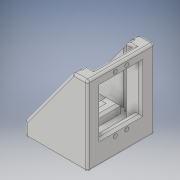
# Autodesk Inventor part: ServoMount2
Saved by Autodesk Inventor 2018 (Build 220112000, 112)
## iProperties
Created: 2018-04-02
Part Number: ServoMount2
Material: Generic
Document SubType Name: Modeling
Designer: anirudh
Density: 1 g/cm^3
Appearance: Default
Author: anirudh
Autodesk Inventor part; units mm, degrees
ref_plane "YZ Plane" through (0, 0, 0) normal (1, 0, 0) x (0, 1, 0)
ref_plane "XZ Plane" through (0, 0, 0) normal (0, 1, 0) x (-1, 0, 0)
ref_plane "XY Plane" through (0, 0, 0) normal (0, 0, 1) x (1, 0, 0)
sketch "Sketch10" plane through (0, 0, 0) normal (0, 1, 0) x (-1, 0, 0)
  line L0 (0, 0) -> (54.4068, 0)
  line L1 (54.4068, 0) -> (54.4068, -58.9534)
  line L2 (54.4068, -58.9534) -> (0, -58.9534)
  line L3 (0, -58.9534) -> (0, 0)
  dimension "d27" = 54.4068
  dimension "d28" = 58.9534
  constraints: 8 end point, 2 parallel, 1 horizontal, 1 perpendicular
  measures "d27" distance of L1.end L2.end
  measures "d28" distance of L0.end L1.end
extrude "Extrusion6" add sketch "Sketch10" along normal blind 76.2
sketch "Sketch12" plane through (0, 0, 0) normal (1, 0, 0) x (0, 0, -1)
  line L0 (58.9534, 0) -> (0, 0) projected
  line L1 (0, 0) -> (58.9534, 0)
  line L2 (58.9534, 0) -> (58.9534, 76.2) projected
  line L3 (0, 0) -> (0, 76.2) projected
  line L4 (29.4767, 20.6375) -> (18.3642, 20.6375)
  line L5 (18.3642, 20.6375) -> (40.5892, 20.6375)
  line L6 (40.5892, 20.6375) -> (40.5892, 60.325)
  line L7 (40.5892, 60.325) -> (18.3642, 60.325)
  line L8 (18.3642, 60.325) -> (18.3642, 20.6375)
  dimension "d39" = 11.1125
  dimension "d40" = 22.225
  constraints: 12 end point, 2 horizontal, 2 parallel, 1 perpendicular
  measures "d39" distance of L4.end L4.start
  measures "d40" distance of L7.end L6.end
extrude "Extrusion7" cut sketch "Sketch12" against normal blind 41.275
sketch "Sketch13" plane through (0, 0, 0) normal (1, 0, 0) x (0, 0, -1)
  line L0 (0, 0) -> (0, 12.7)
  line L1 (0, 12.7) -> (58.9534, 12.7)
  line L2 (0, 68.2752) -> (58.9534, 68.2752)
  line L3 (0, 0) -> (0, 76.2) projected
  line L4 (0, 76.2) -> (58.9534, 76.2)
  line L5 (58.9534, 76.2) -> (58.9534, 68.2752)
  line L6 (58.9534, 68.2752) -> (0, 68.2752)
  line L7 (0, 68.2752) -> (0, 76.2)
  dimension "d43" = 12.7
  constraints: 14 end point, 2 parallel, 2 perpendicular, 1 horizontal
  measures "d43" distance of L0.start L0.end
extrude "Extrusion8" cut sketch "Sketch13" against normal blind 54.4068
sketch "Sketch14" plane through (0, 0, 0) normal (1, 0, 0) x (0, 0, -1)
  line L0 (0, 0) -> (0, 12.7)
  line L1 (0, 0) -> (0, 68.2752) projected
  line L2 (0, 12.7) -> (58.9534, 12.7)
  line L3 (58.9534, 0) -> (58.9534, 68.2752) projected
  line L4 (0, 68.2752) -> (58.9534, 68.2752)
  line L5 (58.9534, 68.2752) -> (58.9534, 12.7)
  line L6 (58.9534, 12.7) -> (0, 12.7)
  line L7 (0, 12.7) -> (0, 68.2752)
  line L8 (18.3642, 60.325) -> (40.5892, 60.325) projected
  line L9 (40.5892, 60.325) -> (40.5892, 20.6375) projected
  line L10 (18.3642, 60.325) -> (40.5892, 60.325)
  line L11 (40.5892, 60.325) -> (40.5892, 20.6375)
  line L12 (40.5892, 20.6375) -> (18.3642, 20.6375)
  line L13 (18.3642, 20.6375) -> (18.3642, 60.325)
  dimension "d47" = 12.7
  constraints: 20 end point, 4 parallel, 3 perpendicular, 2 horizontal, 2 point on line
  measures "d47" distance of L0.start L0.end
extrude "Extrusion9" cut sketch "Sketch14" against normal blind 12.7
sketch "Sketch15" plane through (-54.4068, 0, 0) normal (0, 0, 1) x (1, 0, 0)
  line L0 (41.7068, 12.7) -> (41.7068, 68.2752) projected
  line L1 (0, 0) -> (0, 68.2752) projected
  line L2 (41.7068, 12.7) -> (0, 12.7)
  line L3 (0, 12.7) -> (0, 68.2752)
  line L4 (0, 68.2752) -> (41.7068, 68.2752)
  line L5 (41.7068, 68.2752) -> (41.7068, 12.7)
  point P0 (54.4068, 0)
  constraints: 8 end point, 2 parallel, 1 horizontal, 1 perpendicular
extrude "Extrusion10" cut sketch "Sketch15" against normal blind 12.0142
sketch "Sketch16" plane through (0, 0, -58.9534) normal (0, 0, -1) x (-1, 0, 0)
  line L0 (54.4068, 68.2752) -> (12.7, 68.2752) projected
  line L1 (12.7, 12.7) -> (54.4068, 12.7) projected
  line L2 (12.7, 68.2752) -> (54.4068, 68.2752)
  line L3 (54.4068, 68.2752) -> (54.4068, 12.7)
  line L4 (54.4068, 12.7) -> (12.7, 12.7)
  line L5 (12.7, 12.7) -> (12.7, 68.2752)
  point P0 (0, 0)
  constraints: 8 end point, 2 parallel, 1 horizontal, 1 perpendicular
extrude "Extrusion11" cut sketch "Sketch16" against normal blind 12.0142
sketch "Sketch17" plane through (-54.4068, 0, -58.9534) normal (-1, 0, 0) x (0, 0, 1)
  line L0 (12.0142, 12.7) -> (12.0142, 68.2752) projected
  line L1 (46.9392, 68.2752) -> (46.9392, 12.7) projected
  line L2 (12.0142, 68.2752) -> (46.9392, 68.2752)
  line L3 (46.9392, 68.2752) -> (46.9392, 12.7)
  line L4 (46.9392, 12.7) -> (12.0142, 12.7)
  line L5 (12.0142, 12.7) -> (12.0142, 68.2752)
  point P0 (58.9534, 0)
  constraints: 8 end point, 2 parallel, 1 horizontal, 1 perpendicular
extrude "Extrusion12" cut sketch "Sketch17" against normal blind 6.7818
sketch "Sketch18" plane through (0, 0, 0) normal (0, -1, 0) x (1, 0, 0)
  line L0 (-54.4068, -58.9534) -> (0, -58.9534) projected
  line L1 (0, -58.9534) -> (0, 0) projected
  line L2 (0, 0) -> (-54.4068, 0) projected
  circle A0 centre (-18.034, -52.6034) radius 1.75
  circle A1 centre (-46.7868, -52.6034) radius 1.75
  circle A2 centre (-18.034, -6.35) radius 1.75
  circle A3 centre (-46.7868, -6.35) radius 1.75
  dimension "d61" = 3.5
  dimension "d62" = 3.5
  dimension "d63" = 3.5
  dimension "d64" = 3.5
  constraints: 4 centre point
  measures "d61" diameter of A0
  measures "d62" diameter of A1
  measures "d63" diameter of A2
  measures "d64" diameter of A3
extrude "Extrusion13" cut sketch "Sketch18" against normal blind 12.7
sketch "Sketch21" plane through (-12.7, 0, 0) normal (1, 0, 0) x (0, 0, -1)
  circle A0 centre (24.4348, 64.9986) radius 1.75
  circle A1 centre (34.5186, 64.9986) radius 1.75
  circle A2 centre (24.4348, 15.9639) radius 1.75
  circle A3 centre (34.5186, 15.9639) radius 1.75
  point P0 (0, 0)
  point P1 (18.3642, 20.6375)
  point P2 (18.3642, 60.325)
  dimension "d82" = 3.5
  dimension "d83" = 3.5
  dimension "d84" = 3.5
  dimension "d85" = 3.5
  constraints: 4 centre point
  measures "d82" diameter of A0
  measures "d83" diameter of A1
  measures "d84" diameter of A2
  measures "d85" diameter of A3
extrude "Extrusion15" cut sketch "Sketch21" against normal blind 15.24
sketch "Sketch27" plane through (-12.7, 68.2752, -12.0142) normal (0, 1, 0) x (1, 0, 0)
  line L0 (-28.575, 6.35) -> (-28.575, 28.575) projected
  line L1 (-28.575, 6.35) -> (-5.08, 6.35)
  line L2 (-5.08, 28.575) -> (-28.575, 28.575)
  line L3 (-28.575, 28.575) -> (-28.575, 6.35)
  line L4 (-34.925, 0) -> (-34.925, 34.925) projected
  line L5 (-5.08, 0) -> (-34.925, 0)
  line L6 (-34.925, 0) -> (-34.925, 34.925)
  line L7 (-34.925, 34.925) -> (-5.08, 34.925)
  line L8 (-5.08, 0) -> (-34.925, 0)
  line L9 (-34.925, 0) -> (-34.925, 34.925)
  line L10 (-34.925, 34.925) -> (-5.08, 34.925)
  line L11 (-5.08, 34.925) -> (-5.08, 28.575)
  line L12 (-5.08, 28.575) -> (-28.575, 28.575)
  line L13 (-28.575, 28.575) -> (-28.575, 6.35)
  line L14 (-28.575, 6.35) -> (-5.08, 6.35)
  line L15 (-5.08, 6.35) -> (-5.08, 0)
  point P0 (12.7, -12.0142)
  constraints: 28 end point, 7 equal length, 3 perpendicular, 2 horizontal
extrude "Extrusion18" cut sketch "Sketch27" against normal blind 47.6504
sketch "Sketch28" plane through (-12.7, 68.2752, -12.0142) normal (0, 1, 0) x (1, 0, 0)
  line L0 (-28.575, 28.575) -> (-28.575, 6.35) projected
  line L1 (-5.08, 28.575) -> (-28.575, 28.575) projected
  line L2 (-28.575, 6.35) -> (-5.08, 6.35)
  line L3 (-5.08, 6.35) -> (-5.08, 28.575)
  line L4 (-5.08, 28.575) -> (-28.575, 28.575)
  line L5 (-28.575, 28.575) -> (-28.575, 6.35)
  point P0 (12.7, -12.0142)
  constraints: 8 end point, 2 parallel, 1 horizontal, 1 perpendicular
extrude "Extrusion19" cut sketch "Sketch28" against normal blind 7.9502
sketch "Sketch29" plane through (-12.7, 68.2752, -12.0142) normal (0, 1, 0) x (1, 0, 0)
  line L0 (-5.08, 34.925) -> (-5.08, 28.575) projected
  line L1 (0, 0) -> (-34.925, 0) projected
  line L2 (-5.08, 34.925) -> (0, 34.925)
  line L3 (0, 34.925) -> (0, 0)
  line L4 (0, 0) -> (-5.08, 0)
  line L5 (-5.08, 0) -> (-5.08, 34.925)
  point P0 (12.7, -12.0142)
  constraints: 8 end point, 2 parallel, 1 horizontal, 1 perpendicular
extrude "Extrusion20" add sketch "Sketch29" along normal blind 1.397
sketch "Sketch30" plane through (0, 12.7, 0) normal (0, 1, 0) x (1, 0, 0)
  line L0 (0, 58.9534) -> (0, 0) projected
  line L1 (-54.4068, 58.9534) -> (0, 58.9534) projected
  line L2 (0, 0) -> (-12.7, 0)
  line L3 (-12.7, 0) -> (-12.7, 58.9534)
  line L4 (-12.7, 58.9534) -> (0, 58.9534)
  line L5 (0, 58.9534) -> (0, 0)
  dimension "d117" = 12.7
  constraints: 8 end point, 2 parallel, 1 horizontal, 1 perpendicular, 1 point on line
  measures "d117" distance of L3.end L4.end
extrude "Extrusion21" cut sketch "Sketch30" against normal blind 3.81
sketch "Sketch34" plane through (-12.7, 20.6375, -18.3642) normal (0, 1, 0) x (1, 0, 0)
  line L0 (0, 0) -> (-5.08, 0) projected
  line L1 (-11.43, -6.35) -> (-11.43, 28.575)
  line L2 (-24.13, -6.35) -> (-24.13, 28.575)
  line L3 (-34.925, -6.35) -> (-34.925, 28.575) projected
  line L4 (-24.13, -6.35) -> (-34.925, -6.35)
  line L5 (-34.925, -6.35) -> (-34.925, 28.575)
  line L6 (-34.925, 28.575) -> (-24.13, 28.575)
  line L7 (-24.13, 28.575) -> (-24.13, -6.35)
  line L8 (-11.43, -6.35) -> (-5.08, -6.35)
  line L9 (-5.08, -6.35) -> (-5.08, 28.575)
  line L10 (-5.08, 28.575) -> (-11.43, 28.575)
  line L11 (-11.43, 28.575) -> (-11.43, -6.35)
  point P0 (12.7, -18.3642)
  dimension "d131" = 34.925
  dimension "d132" = 12.7
  constraints: 20 end point, 4 parallel, 2 horizontal, 2 perpendicular
  measures "d131" distance of L1.start L1.end
  measures "d132" distance of L1.start L2.start
extrude "Extrusion25" cut sketch "Sketch34" against normal blind 7.9502
sketch "Sketch35" plane through (0, 8.89, 0) normal (0, 1, 0) x (1, 0, 0)
  line L0 (-12.7, 46.9392) -> (-12.7, 58.9534) projected
  line L1 (0, 58.9534) -> (0, 0) projected
  line L2 (-12.7, 58.9534) -> (0, 58.9534)
  line L3 (0, 58.9534) -> (0, 0)
  line L4 (0, 0) -> (-12.7, 0)
  line L5 (-12.7, 0) -> (-12.7, 58.9534)
  constraints: 8 end point, 2 parallel, 1 horizontal, 1 perpendicular
extrude "Extrusion26" add sketch "Sketch35" along normal blind 11.7602
sketch "Sketch36" plane through (-12.7, 0, 0) normal (1, 0, 0) x (0, 0, -1)
  circle A0 centre (24.4348, 15.9639) radius 1.75 projected
  circle A1 centre (24.4348, 15.9639) radius 1.75
  circle A2 centre (34.5186, 15.9639) radius 1.75 projected
  circle A3 centre (34.5186, 15.9639) radius 1.75
  point P0 (0, 0)
  constraints: 2 centre point, 2 coincident
extrude "Extrusion27" cut sketch "Sketch36" along normal blind 12.7
sketch "Sketch37" plane through (0, 20.6502, 0) normal (0, 1, 0) x (1, 0, 0)
  line L0 (-12.7, 0) -> (-12.7, 12.0142) projected
  line L1 (-12.7, 0) -> (0, 0)
  line L2 (0, 0) -> (0, 12.0142)
  line L3 (0, 12.0142) -> (-12.7, 12.0142)
  line L4 (-12.7, 12.0142) -> (-12.7, 0)
  line L5 (-12.7, 58.9534) -> (-12.7, 46.9392) projected
  line L6 (0, 58.9534) -> (-12.7, 58.9534) projected
  line L7 (-12.7, 46.9392) -> (0, 46.9392)
  line L8 (0, 46.9392) -> (0, 58.9534)
  line L9 (0, 58.9534) -> (-12.7, 58.9534)
  line L10 (-12.7, 58.9534) -> (-12.7, 46.9392)
  constraints: 16 end point, 4 parallel, 2 horizontal, 2 perpendicular
extrude "Extrusion28" add sketch "Sketch37" along normal blind 49.022
sketch "Sketch38" plane through (0, 20.6502, -12.0142) normal (0, 0, -1) x (-1, 0, 0)
  line L0 (0, 0) -> (0, 49.022) projected
  line L1 (12.7, 39.6748) -> (17.78, 39.6748) projected
  line L2 (0, 49.022) -> (12.7, 49.022)
  line L3 (12.7, 49.022) -> (12.7, 39.6748)
  line L4 (12.7, 39.6748) -> (0, 39.6748)
  line L5 (0, 39.6748) -> (0, 49.022)
  point P0 (0, -20.6502)
  constraints: 8 end point, 2 parallel, 1 horizontal, 1 perpendicular
extrude "Extrusion29" add sketch "Sketch38" along normal blind 34.925
sketch "Sketch39" plane through (-12.7, 64.9986, -34.5186) normal (-1, 0, 0) x (0, 0, 1)
  circle A0 centre (0, 0) radius 1.75
  circle A1 centre (10.0838, 0) radius 1.75 projected
  circle A2 centre (10.0838, 0) radius 1.75
  point P0 (34.5186, -64.9986)
  constraints: 2 centre point, 1 coincident
extrude "Extrusion30" cut sketch "Sketch39" against normal blind 12.7
sketch "Sketch40" plane through (-12.7, 69.6722, -12.0142) normal (0, 1, 0) x (1, 0, 0)
  line L0 (0, 0) -> (-5.08, 0) projected
  line L1 (0, 34.925) -> (0, 28.575) projected
  line L2 (-5.08, 0) -> (0, 0)
  line L3 (0, 0) -> (0, 34.925)
  line L4 (0, 34.925) -> (-5.08, 34.925)
  line L5 (-5.08, 34.925) -> (-5.08, 0)
  point P0 (12.7, -12.0142)
  constraints: 8 end point, 2 parallel, 1 horizontal, 1 perpendicular
extrude "Extrusion31" cut sketch "Sketch40" against normal blind 56.9722
sketch "Sketch41" plane through (-12.7, 12.7, -58.9534) normal (-1, 0, 0) x (0, 0, 1)
  line L0 (46.9392, 47.625) -> (12.0142, 47.625) projected
  line L1 (58.9534, 56.9722) -> (0, 56.9722) projected
  line L2 (12.0142, 47.625) -> (46.9392, 47.625)
  line L3 (46.9392, 47.625) -> (46.9392, 56.9722)
  line L4 (46.9392, 56.9722) -> (12.0142, 56.9722)
  line L5 (12.0142, 56.9722) -> (12.0142, 47.625)
  line L6 (0, 0) -> (58.9534, 0) projected
  line L7 (12.0142, 7.9502) -> (46.9392, 7.9502)
  line L8 (46.9392, 7.9502) -> (46.9392, 0)
  line L9 (46.9392, 0) -> (12.0142, 0)
  line L10 (12.0142, 0) -> (12.0142, 7.9502)
  circle A0 centre (24.4348, 52.2986) radius 1.75 projected
  circle A1 centre (24.4348, 52.2986) radius 1.75
  circle A2 centre (34.5186, 52.2986) radius 1.75 projected
  circle A3 centre (34.5186, 52.2986) radius 1.75
  circle A4 centre (24.4348, 3.2639) radius 1.75 projected
  circle A5 centre (24.4348, 3.2639) radius 1.75
  circle A6 centre (34.5186, 3.2639) radius 1.75 projected
  circle A7 centre (34.5186, 3.2639) radius 1.75
  point P0 (58.9534, -12.7)
  dimension "d148" = 34.925
  constraints: 16 end point, 4 centre point, 4 coincident, 4 parallel, 2 horizontal, 2 perpendicular, 2 point on line
  measures "d148" distance of L4.end L3.end
extrude "Extrusion32" cut sketch "Sketch41" against normal blind 6.35
sketch "Sketch42" plane through (-24.13, 20.6375, -18.3642) normal (1, 0, 0) x (0, 0, -1)
  line L0 (-6.35, -0.0127) -> (0, -0.0127) projected
  line L1 (-6.35, -0.0127) -> (28.575, -0.0127)
  line L2 (28.575, -0.0127) -> (28.575, -7.9502)
  line L3 (28.575, -7.9502) -> (-6.35, -7.9502)
  line L4 (-6.35, -7.9502) -> (-6.35, -0.0127)
  point P0 (-18.3642, -20.6375)
  constraints: 8 end point, 2 parallel, 1 horizontal, 1 perpendicular
extrude "Extrusion33" add sketch "Sketch42" along normal blind 6.35
sketch "Sketch43" plane through (-36.83, 20.6375, -40.5892) normal (-1, 0, 0) x (0, 0, 1)
  line L0 (-6.35, -7.9375) -> (-6.35, 0.0127) projected
  line L1 (28.575, -7.9375) -> (-6.35, -7.9375) projected
  line L2 (-6.35, 0.0127) -> (28.575, 0.0127)
  line L3 (28.575, 0.0127) -> (28.575, -7.9375)
  line L4 (28.575, -7.9375) -> (-6.35, -7.9375)
  line L5 (-6.35, -7.9375) -> (-6.35, 0.0127)
  point P0 (40.5892, -20.6375)
  constraints: 8 end point, 2 parallel, 1 horizontal, 1 perpendicular
extrude "Extrusion34" cut sketch "Sketch43" against normal blind 6.35
sketch "Sketch45" plane through (0, 0, -58.9534) normal (0, 0, -1) x (-1, 0, 0)
  line L0 (12.7, 12.7) -> (6.35, 12.7) projected
  line L1 (12.7, 69.6722) -> (12.7, 12.7)
  line L2 (12.7, 12.7) -> (54.4068, 12.7) projected
  line L3 (12.7, 12.7) -> (54.4068, 12.7)
  line L4 (54.4068, 12.7) -> (12.7, 69.6722)
  point P0 (0, 0)
  constraints: 6 end point, 1 collinear, 1 vertical
extrude "Extrusion35" add sketch "Sketch45" against normal blind 6.35
sketch "Sketch46" plane through (-54.4068, 0, 0) normal (0, 0, 1) x (1, 0, 0)
  line L0 (41.7068, 69.6722) -> (41.7068, 12.7) projected
  line L1 (41.7068, 69.6722) -> (41.7068, 12.7)
  line L2 (41.7068, 69.6722) -> (0, 12.7) projected
  line L3 (41.7068, 12.7) -> (0, 12.7)
  point P0 (54.4068, 0)
  constraints: 4 end point, 1 collinear, 1 perpendicular
extrude "Extrusion36" add sketch "Sketch46" against normal blind 6.35
sketch "Sketch48" plane through (0, 0, 0) normal (0, -1, 0) x (1, 0, 0)
  circle A0 centre (-46.7868, -52.6034) radius 1.75 projected
  circle A1 centre (-46.7868, -52.6034) radius 1.75
  circle A2 centre (-46.7868, -6.35) radius 1.75 projected
  circle A3 centre (-46.7868, -6.35) radius 1.75
  circle A4 centre (-18.034, -6.35) radius 1.75 projected
  circle A5 centre (-18.034, -6.35) radius 1.75
  circle A6 centre (-18.034, -52.6034) radius 1.75 projected
  circle A7 centre (-18.034, -52.6034) radius 1.75
  point P0 (0, 0)
  constraints: 4 centre point, 4 coincident
hole "Hole1" at (-46.7868, 0, -52.6034) at (-46.7868, 0, -6.35) at (-18.034, 0, -6.35) at (-18.034, 0, -52.6034) direction (0, 1, 0) diameter 3.5 depth 57.15 tip angle 118
sketch "Sketch49" plane through (-12.7, 12.7, -12.0142) normal (0, 1, 0) x (1, 0, 0)
  circle A0 centre (-34.0868, 40.5892) radius 1.75 projected
  circle A1 centre (-34.0868, 40.5892) radius 1.75
  circle A2 centre (-5.334, 40.5892) radius 1.75 projected
  circle A3 centre (-5.334, 40.5892) radius 1.75
  circle A4 centre (-5.334, -5.6642) radius 1.75 projected
  circle A5 centre (-5.334, -5.6642) radius 1.75
  circle A6 centre (-34.0868, -5.6642) radius 1.75 projected
  circle A7 centre (-34.0868, -5.6642) radius 1.75
  point P0 (12.7, -12.0142)
  constraints: 4 centre point, 4 coincident
hole "Hole2" at (-18.034, 12.7, -52.6034) at (-46.7868, 12.7, -52.6034) at (-18.034, 12.7, -6.35) at (-46.7868, 12.7, -6.35) direction (0, 1, 0) diameter 6.35 depth 56.9722 tip angle 118
fillet "Fillet5" radius 1.905 13 edges at (-33.5534, 41.1861, -58.9534) (-6.35, 69.6722, -58.9534) (0, 34.8361, -58.9534) (-27.2034, 0, -58.9534) (-54.4068, 6.35, -58.9534) (0, 0, -29.4767) (0, 34.8361, 0) (0, 69.6722, -29.4767) (-33.5534, 41.1861, 0) (-6.35, 69.6722, 0) (-54.4068, 6.35, 0) (-27.2034, 0, 0) (-54.4068, 0, -29.4767)
chamfer "Chamfer5" distance 1.905 angle 45 9 edges at (-30.48, 20.6375, -29.4767) (-24.13, 20.6248, -46.9392) (-17.78, 20.6248, -29.4767) (-24.13, 20.6248, -12.0142) (0, 40.4876, -12.0142) (0, 20.6502, -29.4767) (-6.35, 20.6502, -29.4767) (0, 40.4876, -46.9392) (0, 60.325, -29.4767)
fillet "Fillet6" radius 1.905 9 edges at (-9.525, 69.6722, -12.0142) (-12.7, 69.6722, -9.1821) (-6.35, 69.6722, -29.4767) (-12.7, 69.6722, -49.7713) (-9.525, 69.6722, -46.9392) (-12.7, 69.6722, -54.8259) (-12.417, 69.1142, -58.3954) (-12.417, 69.1142, -0.558) (-12.7, 69.6722, -4.1275)
body "Solid2"
